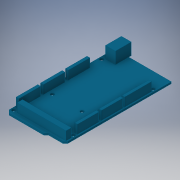
# Autodesk Inventor part: Arduino Due
Saved by Autodesk Inventor 2018 (Build 220112000, 112)
## iProperties
Created: 2021-03-23
Part Number: Arduino Due
Material: Generic
Document SubType Name: Modeling
Designer: Charles.Rymal
Density: 1 g/cm^3
Appearance: Default
Author: Charles.Rymal
Autodesk Inventor part; units mm, degrees
ref_plane "YZ Plane" through (0, 0, 0) normal (1, 0, 0) x (0, 1, 0)
ref_plane "XZ Plane" through (0, 0, 0) normal (0, 1, 0) x (-1, 0, 0)
ref_plane "XY Plane" through (0, 0, 0) normal (0, 0, 1) x (1, 0, 0)
sketch "Sketch1" plane through (0, 0, 0) normal (0, 1, 0) x (-1, 0, 0)
  line L0 (-26.605, -50.8) -> (26.605, -50.8)
  line L1 (26.605, -50.8) -> (26.605, 48.05)
  line L2 (23.855, 50.8) -> (-8.395, 50.8)
  line L3 (-26.605, 46.3) -> (-26.605, -50.8)
  line L4 (26.605, 48.05) -> (23.855, 50.8)
  line L5 (-8.395, 50.8) -> (-10.645, 48.55)
  line L6 (-10.645, 48.55) -> (-24.355, 48.55)
  line L7 (-24.355, 48.55) -> (-26.605, 46.3)
  circle A0 centre (24.065, -36.2) radius 1.59
  circle A1 centre (18.855, 15.3) radius 1.59
  circle A2 centre (-24.195, 38.73) radius 1.59
  circle A3 centre (24.065, 46.35) radius 1.59
  circle A4 centre (-8.995, 15.3) radius 1.59
  circle A5 centre (-24.195, -36.2) radius 1.59
  line L8 (24.065, -36.2) -> (24.065, 46.35) construction
  line L9 (24.065, -36.2) -> (-24.195, -36.2) construction
  line L10 (-24.195, -36.2) -> (-24.195, 38.73) construction
  line L11 (18.855, 15.3) -> (-8.995, 15.3) construction
  point P0 (0, 0)
  dimension "d4" = 2.25
  dimension "d5" = 45
  dimension "d6" = 2.25
  dimension "d7" = 45
  dimension "d8" = 2.75
  dimension "d9" = 35
  dimension "d10" = 53.21
  dimension "d11" = 101.6
  dimension "d12" = 50.8
  dimension "d13" = 26.605
  dimension "d14" = 2.54
  dimension "d15" = 7.75
  dimension "d16" = 82.55
  dimension "d17" = 74.93
  dimension "d18" = 48.26
  dimension "d19" = 66.1
  dimension "d20" = 3.18
  dimension "d21" = 27.85
  dimension "d22" = 14.6
  constraints: 24 end point, 6 centre point, 5 equal radius, 4 horizontal, 3 parallel, 2 vertical, 1 perpendicular
  measures "d4" distance between parallel lines of L2 L6
  measures "d5" angle of L3 L7
  measures "d6" distance from line of L3.start L6
  measures "d7" angle of L2 L4
  measures "d8" distance from line of L1.end L2
  measures "d9" distance from line of L2.end L1
  measures "d10" distance between parallel lines of L1 L3
  measures "d11" distance between parallel lines of L0 L2
  measures "d12" distance from line of point (0, 0) L0
  measures "d13" distance from line of L3 point (0, 0)
  measures "d14" distance between parallel lines of L1 L8
  measures "d15" distance from line of L11.start L1
  measures "d16" distance from line of L9 L8.end
  measures "d17" distance of L9.end L10.end
  measures "d18" distance of L8.start L9.end
  measures "d19" distance between parallel lines of L11 L0
  measures "d20" diameter of A0
  measures "d21" distance of L11.start L11.end
  measures "d22" distance between parallel lines of L9 L0
extrude "Extrusion1" add sketch "Sketch1" against normal blind 1.65
sketch "Sketch2" plane through (0, 0, 0) normal (0, 1, 0) x (1, 0, 0)
  circle A0 centre (24.195, 36.2) radius 1.59 projected
  circle A1 centre (8.995, -15.3) radius 1.59 projected
  circle A2 centre (-24.065, -46.35) radius 1.59 projected
  circle A3 centre (24.195, -38.73) radius 1.59 projected
  circle A4 centre (-18.855, -15.3) radius 1.59 projected
  circle A5 centre (-24.065, 36.2) radius 1.59 projected
  line L0 (26.605, 50.8) -> (-26.605, 50.8) projected
  line L1 (-26.605, 50.8) -> (-26.605, -48.05) projected
  line L2 (-26.605, -48.05) -> (-23.855, -50.8) projected
  line L3 (-23.855, -50.8) -> (8.395, -50.8) projected
  line L4 (8.395, -50.8) -> (10.645, -48.55) projected
  line L5 (10.645, -48.55) -> (24.355, -48.55) projected
  line L6 (24.355, -48.55) -> (26.605, -46.3) projected
  line L7 (26.605, -46.3) -> (26.605, 50.8) projected
  circle A6 centre (24.195, 36.2) radius 1.59 projected
  line L8 (24.195, 36.2) -> (24.195, -38.73) construction
  line L9 (25.445, 7.9669) -> (22.945, 7.9669)
  line L10 (22.945, 7.9669) -> (22.945, 33.3669)
  line L11 (22.945, 33.3669) -> (25.445, 33.3669)
  line L12 (25.445, 33.3669) -> (25.445, 7.9669)
  line L13 (25.445, 7.9669) -> (22.945, 33.3669) construction
  line L14 (22.945, 7.9669) -> (25.445, 33.3669) construction
  line L15 (22.945, -13.6564) -> (25.445, -13.6564)
  line L16 (25.445, -13.6564) -> (25.445, 6.6636)
  line L17 (25.445, 6.6636) -> (22.945, 6.6636)
  line L18 (22.945, 6.6636) -> (22.945, -13.6564)
  line L19 (22.945, -13.6564) -> (25.445, 6.6636) construction
  line L20 (25.445, -13.6564) -> (22.945, 6.6636) construction
  line L21 (22.945, -36.2234) -> (25.445, -36.2234)
  line L22 (25.445, -36.2234) -> (25.445, -15.9034)
  line L23 (25.445, -15.9034) -> (22.945, -15.9034)
  line L24 (22.945, -15.9034) -> (22.945, -36.2234)
  line L25 (22.945, -36.2234) -> (25.445, -15.9034) construction
  line L26 (25.445, -36.2234) -> (22.945, -15.9034) construction
  line L27 (-20.3658, -46.7367) -> (25.3542, -46.7367)
  line L28 (25.3542, -46.7367) -> (25.3542, -41.7367)
  line L29 (25.3542, -41.7367) -> (-20.3658, -41.7367)
  line L30 (-20.3658, -41.7367) -> (-20.3658, -46.7367)
  line L31 (-20.3658, -46.7367) -> (25.3542, -41.7367) construction
  line L32 (25.3542, -46.7367) -> (-20.3658, -41.7367) construction
  circle A7 centre (-24.065, 36.2) radius 1.59 projected
  line L33 (-24.065, 36.2) -> (-24.065, -46.35) construction
  line L34 (-25.315, 3.37) -> (-22.815, 3.37)
  line L35 (-22.815, 3.37) -> (-22.815, 23.69)
  line L36 (-22.815, 23.69) -> (-25.315, 23.69)
  line L37 (-25.315, 23.69) -> (-25.315, 3.37)
  line L38 (-25.315, 3.37) -> (-22.815, 23.69) construction
  line L39 (-22.815, 3.37) -> (-25.315, 23.69) construction
  line L40 (-25.315, -19.9342) -> (-22.815, -19.9342)
  line L41 (-22.815, -19.9342) -> (-22.815, 0.3858)
  line L42 (-22.815, 0.3858) -> (-25.315, 0.3858)
  line L43 (-25.315, 0.3858) -> (-25.315, -19.9342)
  line L44 (-25.315, -19.9342) -> (-22.815, 0.3858) construction
  line L45 (-22.815, -19.9342) -> (-25.315, 0.3858) construction
  line L46 (-25.315, -42.7584) -> (-22.815, -42.7584)
  line L47 (-22.815, -42.7584) -> (-22.815, -22.4384)
  line L48 (-22.815, -22.4384) -> (-25.315, -22.4384)
  line L49 (-25.315, -22.4384) -> (-25.315, -42.7584)
  line L50 (-25.315, -42.7584) -> (-22.815, -22.4384) construction
  line L51 (-22.815, -42.7584) -> (-25.315, -22.4384) construction
  point P0 (0, 0)
  point P1 (24.195, 20.6669)
  point P2 (24.195, -3.4964)
  point P3 (24.195, -26.0634)
  point P4 (2.4942, -44.2367)
  point P5 (-24.065, 13.53)
  point P6 (-24.065, -9.7742)
  point P7 (-24.065, -32.5984)
  dimension "d23" = 25.4
  dimension "d24" = 20.32
  dimension "d25" = 2.5
  dimension "d26" = 20.32
  dimension "d27" = 5
  dimension "d28" = 45.72
  dimension "d29" = 20.32
  dimension "d30" = 20.32
  dimension "d31" = 20.32
  constraints: 88 end point, 16 parallel, 14 midpoint, 9 point on line, 7 horizontal, 7 perpendicular, 2 vertical
  measures "d23" distance of L11.end L9.start
  measures "d24" distance of L15.end L16.end
  measures "d25" distance between parallel lines of L10 L12
  measures "d26" distance of L21.end L22.end
  measures "d27" distance of L27.end L28.end
  measures "d28" distance of L27.start L27.end
  measures "d29" distance of L36.end L34.start
  measures "d30" distance of L42.end L40.start
  measures "d31" distance of L48.end L46.start
extrude "Extrusion2" add sketch "Sketch2" along normal blind 8.3 contours L9 L10 L11 L12 | L18 L17 L16 L15 | L24 L23 L22 L21 | L30 L29 L28 L27 | L37 L36 L35 L34 | L43 L42 L41 L40 | L49 L48 L47 L46
sketch "Sketch3" plane through (0, 0, 0) normal (0, 1, 0) x (1, 0, 0)
  line L0 (22.945, 7.9669) -> (22.945, 33.3669) projected
  line L1 (22.945, 33.3669) -> (25.445, 33.3669) projected
  line L2 (25.445, 33.3669) -> (25.445, 7.9669) projected
  line L3 (25.445, 7.9669) -> (22.945, 7.9669) projected
  line L4 (-25.315, -19.9342) -> (-25.315, 0.3858) projected
  line L5 (-25.315, 0.3858) -> (-22.815, 0.3858) projected
  line L6 (-22.815, 0.3858) -> (-22.815, -19.9342) projected
  line L7 (-22.815, -19.9342) -> (-25.315, -19.9342) projected
  line L8 (22.945, -36.2234) -> (22.945, -15.9034) projected
  line L9 (22.945, -15.9034) -> (25.445, -15.9034) projected
  line L10 (25.445, -15.9034) -> (25.445, -36.2234) projected
  line L11 (25.445, -36.2234) -> (22.945, -36.2234) projected
  line L12 (22.945, -13.6564) -> (22.945, 6.6636) projected
  line L13 (22.945, 6.6636) -> (25.445, 6.6636) projected
  line L14 (25.445, 6.6636) -> (25.445, -13.6564) projected
  line L15 (25.445, -13.6564) -> (22.945, -13.6564) projected
  line L16 (-25.315, 3.37) -> (-25.315, 23.69) projected
  line L17 (-25.315, 23.69) -> (-22.815, 23.69) projected
  line L18 (-22.815, 23.69) -> (-22.815, 3.37) projected
  line L19 (-22.815, 3.37) -> (-25.315, 3.37) projected
  line L20 (-25.315, -42.7584) -> (-25.315, -22.4384) projected
  line L21 (-25.315, -22.4384) -> (-22.815, -22.4384) projected
  line L22 (-22.815, -22.4384) -> (-22.815, -42.7584) projected
  line L23 (-22.815, -42.7584) -> (-25.315, -42.7584) projected
  line L24 (-20.3658, -46.7367) -> (-20.3658, -41.7367) projected
  line L25 (-20.3658, -41.7367) -> (25.3542, -41.7367) projected
  line L26 (25.3542, -41.7367) -> (25.3542, -46.7367) projected
  line L27 (25.3542, -46.7367) -> (-20.3658, -46.7367) projected
  circle A0 centre (24.195, 36.2) radius 1.59 projected
  circle A1 centre (8.995, -15.3) radius 1.59 projected
  circle A2 centre (-24.065, -46.35) radius 1.59 projected
  circle A3 centre (24.195, -38.73) radius 1.59 projected
  circle A4 centre (-18.855, -15.3) radius 1.59 projected
  circle A5 centre (-24.065, 36.2) radius 1.59 projected
  line L28 (26.605, 50.8) -> (-26.605, 50.8) projected
  line L29 (-26.605, 50.8) -> (-26.605, -48.05) projected
  line L30 (-26.605, -48.05) -> (-23.855, -50.8) projected
  line L31 (-23.855, -50.8) -> (8.395, -50.8) projected
  line L32 (8.395, -50.8) -> (10.645, -48.55) projected
  line L33 (10.645, -48.55) -> (24.355, -48.55) projected
  line L34 (24.355, -48.55) -> (26.605, -46.3) projected
  line L35 (26.605, -46.3) -> (26.605, 50.8) projected
  line L36 (-13.335, 53.1213) -> (-22.475, 53.1213)
  line L37 (-22.475, 53.1213) -> (-22.475, 38.2805)
  line L38 (-22.475, 38.2805) -> (-13.335, 38.2805)
  line L39 (-13.335, 38.2805) -> (-13.335, 53.1213)
  point P0 (0, 0)
  dimension "d34" = 9.14
  constraints: 8 end point, 2 parallel, 1 horizontal, 1 perpendicular
  measures "d34" distance of L36.start L36.end
extrude "Extrusion3" add sketch "Sketch3" along normal blind 11.18 contours L39 L38 L37 L28 | L28 L37 L36 L39
body "Solid1"
